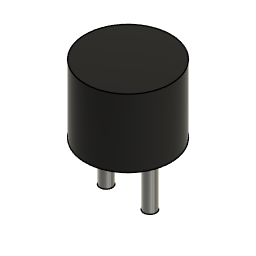
BabyRoboting (Autodesk Fusion 360 archive; units mm, degrees)
design "PassiveBuzzer"
Autodesk Fusion 360 part; units mm, degrees
sketch "Sketch1" plane through (0, 0, 0) normal (0, 0, 1) x (1, 0, 0)
  circle A0 centre (0, 0) radius 5.85
  dimension "d1" = 11.7
  constraint coincident A0.centre origin
  measures "d1" diameter of A0
extrude "Extrude1" add sketch "Sketch1" along normal blind 9.3
sketch "Sketch2" plane through (0, 0, 0) normal (0, 0, -1) x (1, 0, 0)
  circle A0 centre (0, 0) radius 5.85
  circle A1 centre (3, 0) radius 0.85
  line L0 (0, 0) -> (-5.85, 0)
  line L1 (0, 0) -> (5.85, 0)
  line L2 (0, 0) -> (0, 5.85)
  line L3 (0, 0) -> (0, -5.85)
  circle A2 centre (-3, 0) radius 0.85
  dimension "d4" = 1.7
  dimension "d5" = 3
  constraint coincident A0.centre L0.start
  constraint coincident A0 L0.end
  constraint horizontal L0
  constraint coincident A0 L1.end
  constraint parallel L0 L1
  constraint coincident A1.centre L1
  constraint coincident A0 L2.end
  constraint perpendicular L1 L2
  constraint coincident A0 L3.end
  constraint perpendicular L1 L3
  constraint symmetric A1 L2 A2
  measures "d4" diameter of A1
  measures "d5" distance of A0.centre A1.centre
extrude "Extrude2" add sketch "Sketch2" along normal blind 7 contours A1 L1 | A1 L1 | L0 A2 | L0 A2

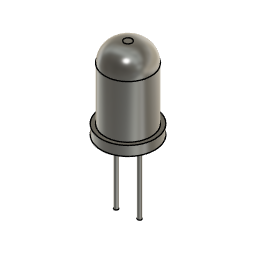
design "LED 5mm"
Autodesk Fusion 360 part; units mm, degrees
sketch "Sketch1" plane through (0, 0, 0) normal (0, 0, 1) x (1, 0, 0)
  circle A0 centre (0, 0) radius 2.4
  circle A1 centre (0, 0) radius 2.8
  dimension "d1" = 4.8
  dimension "d2" = 0.4
  constraint coincident A0.centre A1.centre
  measures "d1" diameter of A0
extrude "Extrude1" add sketch "Sketch1" along normal blind 8.5 contours A0
extrude "Extrude2" add sketch "Sketch1" along normal blind 1
fillet "Fillet1" radius 2 1 edges at (-2.2376, -0.8679, 8.5)
sketch "Sketch2" plane through (0, 0, 0) normal (0, 0, 1) x (1, 0, 0)
  circle A0 centre (1.2227, -0.0137) radius 0.2
  line L0 (0, -2.8) -> (0, 2.8)
  circle A1 centre (-1.2227, -0.0137) radius 0.2
  point P0 (-1.2227, -0.0137)
  dimension "d9" = 0.4
  constraint vertical L0
  constraint symmetric A0.centre L0 P0
  constraint symmetric A0 L0 A1
  measures "d9" diameter of A0
extrude "Extrude3" add sketch "Sketch2" against normal blind 7 contours A0
extrude "Extrude4" add sketch "Sketch2" against normal blind 7.3 contours A1
